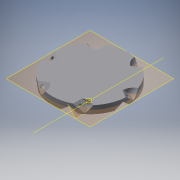
# Autodesk Inventor part: CheekPlate
Saved by Autodesk Inventor 2018 (Build 220112000, 112)
## iProperties
Created: 2017-09-05
Part Number: CheekPlate
Material: Generic
Document SubType Name: Modeling
Designer: P136265
Density: 1 g/cm^3
Appearance: Default
Author: P136265
Autodesk Inventor part; units mm, degrees
ref_plane "YZ Plane" through (0, 0, 0) normal (1, 0, 0) x (0, 1, 0)
ref_plane "XZ Plane" through (0, 0, 0) normal (0, 1, 0) x (-1, 0, 0)
ref_plane "Work Plane1" through (0, 0, 47.5) normal (0, 0, 1) x (1, 0, 0)
sketch "Sketch1" plane through (0, 0, 47.5) normal (0, 0, 1) x (1, 0, 0)
  circle A0 centre (0, 0) radius 97
  dimension "d1" = 194
  constraints: 1 centre point, 1 coincident
  measures "d1" diameter of A0
extrude "Extrusion1" add sketch "Sketch1" along normal mid plane 20
ref_plane "Work Plane8" through (43.4971, -89.2355, 43.4971) normal (0.7071068, 0, 0.7071068) x (0, 1, 0)
sketch "Sketch3" plane through (43.4971, -89.2355, 43.4971) normal (0.7071068, 0, 0.7071068) x (0, 1, 0)
  point P0 (89.2355, 0)
ref_plane "Work Plane9" through (0, 0, 0) normal (0.7071068, 0, -0.7071068) x (0, 1, 0)
sketch "Sketch4" plane through (0, 0, 0) normal (0.7071068, 0, -0.7071068) x (0, 1, 0)
  spline S0 degree 3 poles (-89.2355, -61.5142) (-90.3927, -58.6064) (-92.539, -52.544) (-94.7745, -44.4386) (-96.6571, -36.0105) (-97.8745, -29.0401) (-99.0232, -20.1209) (-99.6396, -12.8528) (-100.0257, -3.6842) (-100.0257, 3.6842) (-99.6396, 12.8528) (-99.0232, 20.1209) (-97.8745, 29.0401) (-96.6571, 36.0105) (-94.7745, 44.4386) (-92.539, 52.544) (-90.3927, 58.6064) (-89.2355, 61.5142) knots 4.04016 4.04016 4.04016 4.04016 4.152198 4.264236 4.320255 4.432293 4.488313 4.600351 4.65637 4.768408 4.824427 4.936465 4.992485 5.104523 5.160542 5.27258 5.384618 5.384618 5.384618 5.384618 construction
  line L0 (-89.2355, 61.5142) -> (-60.7645, 61.5142) construction
  line L1 (-89.2355, -61.5142) -> (-60.7645, -61.5142) construction
  line L2 (-75, 61.5142) -> (-75, 62.5142) construction
  line L3 (-75, 62.5142) -> (-89.2355, 62.5142)
  line L4 (-89.2355, 62.5142) -> (-92.2355, 62.5142)
  line L5 (-75, -61.5142) -> (-75, -62.5142) construction
  line L6 (-75, -62.5142) -> (-89.2355, -62.5142)
  line L7 (-89.2355, -62.5142) -> (-92.2355, -62.5142)
  line L8 (-75, 62.5142) -> (-75, -62.5142)
  line L9 (-75, 0) -> (-103, 0) construction
  arc A0 (-103, 0) -> (-92.2355, -62.5142) centre (83.9064, 0) ccw
  arc A1 (-92.2355, 62.5142) -> (-103, 0) centre (83.9064, 0) ccw
  point P0 (0, 0)
  dimension "d5" = 1
  dimension "d6" = 3
  dimension "d7" = 1
  dimension "d8" = 3
  dimension "d9" = 28
  dimension "d11" = 186.9064
  constraints: 16 end point, 4 point on circle, 3 midpoint, 2 centre point, 2 perpendicular, 2 point on line, 2 vertical, 1 horizontal, 1 parallel, 1 other
  measures "d5" distance of L2.start L2.end
  measures "d6" distance of L3.end L4.end
  measures "d7" distance of L5.start L5.end
  measures "d8" distance of L7.end L6.end
  measures "d9" distance of L9.start L9.end
  measures "d11" radius of A1
revolve "Revolution1" cut sketch "Sketch4" angle 360 about axis through (44.2042, -75, 44.2042) along (-0.7071068, 0, -0.7071068)
ref_plane "Work Plane10" through (71.7613, -75, 71.7613) normal (0.7071068, 0, 0.7071068) x (-0.2977096, -0.9070491, 0.2977096)
sketch "Sketch5" plane through (71.7613, -75, 71.7613) normal (0.7071068, 0, 0.7071068) x (-0.2977096, -0.9070491, 0.2977096)
  circle A0 centre (0, 0) radius 3.5 construction
  circle A1 centre (0, 0) radius 15
  point P0 (-68.0287, -31.5769)
  dimension "d14" = 30
  constraints: 1 centre point, 1 coincident
  measures "d14" diameter of A1
extrude "Extrusion2" cut sketch "Sketch5" against normal blind 30
sketch "Sketch6" plane through (50.5481, -75, 50.5481) normal (0.7071068, 0, 0.7071068) x (0.6413805, -0.421025, -0.6413805)
  circle A0 centre (0, 0) radius 4 construction
  circle A1 centre (0, 0) radius 4.25
  point P0 (-31.5769, 68.0287)
  dimension "d17" = 8.5
  constraints: 1 centre point, 1 coincident
  measures "d17" diameter of A1
extrude "Extrusion3" cut sketch "Sketch6" against normal blind 10
pattern_circular "Circular Pattern1" count 6 over 360 about axis through (0, 0, 47.5) along (0, 0, 1) of "Extrusion2"
pattern_circular "Circular Pattern2" count 6 over 360 about axis through (0, 0, 47.5) along (0, 0, 1) of "Extrusion3"
pattern_circular "Circular Pattern3" count 6 over 360 about axis through (0, 0, 47.5) along (0, 0, 1) of "Revolution1"
body "Solid1"
